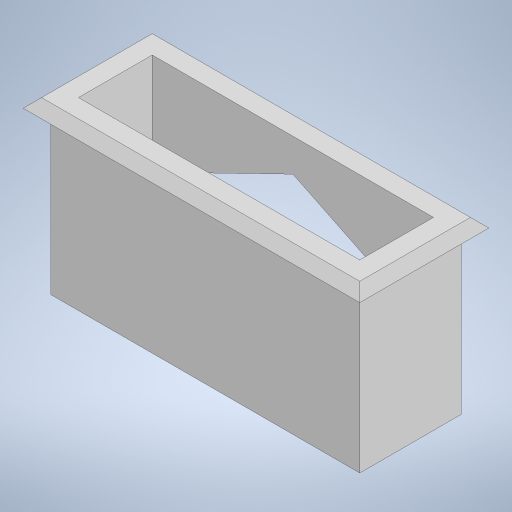
# Autodesk Inventor part: Controller Stand Breakout Holder
Saved by Autodesk Inventor 2024.1 (Build 281209000, 209)
## iProperties
Created: 2024-02-12
Part Number: Controller Stand Breakout Holder
Material: Generic
Document SubType Name: Modeling
Designer: ryanm
Density: 1 g/cm^3
Appearance: Default
Author: ryanm
Autodesk Inventor part; units mm, degrees
ref_plane "YZ Plane" through (0, 0, 0) normal (1, 0, 0) x (0, 1, 0)
ref_plane "XZ Plane" through (0, 0, 0) normal (0, 1, 0) x (-1, 0, 0)
ref_plane "XY Plane" through (0, 0, 0) normal (0, 0, 1) x (1, 0, 0)
sketch "Sketch1" plane through (0, 0, 0) normal (0, 1, 0) x (-1, 0, 0)
  line L0 (30.5, -8) -> (-30.5, -8)
  line L1 (-30.5, -8) -> (-30.5, 8)
  line L2 (-30.5, 8) -> (30.5, 8)
  line L3 (30.5, 8) -> (30.5, -8)
  line L4 (33.5, -11) -> (-33.5, -11)
  line L5 (-33.5, -11) -> (-33.5, 11)
  line L6 (-33.5, 11) -> (33.5, 11)
  line L7 (33.5, 11) -> (33.5, -11)
  point P0 (0, 0)
  point P1 (0, -8)
  point P2 (30.5, 0)
  dimension "d0" = 16
  dimension "d2" = 3
  dimension "d3" = 61
  constraints: 16 end point, 4 parallel, 2 midpoint, 2 perpendicular, 1 horizontal, 1 horizontal alignment, 1 vertical alignment, 3 other
  measures "d0" distance of L2.end L0.start
  measures "d2" distance between parallel lines of L3 L7
  measures "d3" distance of L0.start L0.end
extrude "Extrusion1" add sketch "Sketch1" along normal blind 35
sketch "Sketch2" plane through (0, 35, 0) normal (0, 1, 0) x (1, 0, 0)
  line L0 (-30.5, -8) -> (-30.5, 8) projected
  line L1 (30.5, -8) -> (-30.5, -8) projected
  line L2 (30.5, 8) -> (30.5, -8) projected
  line L3 (-30.5, 8) -> (30.5, 8) projected
  line L4 (-36.5, 14) -> (-36.5, -14)
  line L5 (-36.5, -14) -> (36.5, -14)
  line L6 (36.5, -14) -> (36.5, 14)
  line L7 (36.5, 14) -> (-36.5, 14)
  point P0 (0, 0)
  dimension "d6" = 6
  constraints: 8 end point, 3 other
  measures "d6" distance between parallel lines of L0 L4
extrude "Extrusion2" add sketch "Sketch2" along normal blind 2
chamfer "Chamfer1" distance 2 angle 45 4 edges at (0, 37, 14) (-36.5, 37, 0) (0, 37, -14) (36.5, 37, 0)
sketch "Sketch3" plane through (-30.5, 0, 8) normal (1, 0, 0) x (0, 0, -1)
  line L0 (19, 0) -> (-3, 0) projected
  line L1 (-3, 0) -> (-3, 35) projected
  line L2 (19, 35) -> (-3, 35) projected
  line L3 (19, 0) -> (19, 35) projected
  line L4 (0, 0) -> (2, 0)
  line L5 (2, 0) -> (2, 23)
  line L6 (2, 23) -> (0, 23)
  line L7 (0, 23) -> (0, 0)
  line L8 (4.5, 0) -> (6.5, 0)
  line L9 (6.5, 0) -> (6.5, 12)
  line L10 (6.5, 12) -> (4.5, 12)
  line L11 (4.5, 12) -> (4.5, 0)
  point P0 (8, 0)
  point P1 (2, 0)
  dimension "d12" = 2
  dimension "d13" = 3
  dimension "d14" = 23
  dimension "d28" = 12
  dimension "d29" = 2
  dimension "d30" = 2.5
  constraints: 16 end point, 4 parallel, 2 horizontal, 2 perpendicular, 2 point on line
  measures "d12" distance of L6.end L5.end
  measures "d13" distance between parallel lines of L1 L7
  measures "d14" distance of L4.end L5.end
  measures "d28" distance of L8.end L9.end
  measures "d29" distance of L9.end L10.end
  measures "d30" distance between parallel lines of L5 L11
extrude "Extrusion3" add sketch "Sketch3" along normal blind 2 contours L0 L11 L10 L9 | L0 L7 L6 L5
sketch "Sketch4" plane through (30.5, 0, -8) normal (-1, 0, 0) x (0, 0, 1)
  line L0 (19, 0) -> (-3, 0) projected
  line L1 (-3, 0) -> (-3, 35) projected
  line L2 (19, 35) -> (-3, 35) projected
  line L3 (19, 0) -> (19, 35) projected
  line L4 (14, 0) -> (16, 0)
  line L5 (16, 0) -> (16, 23)
  line L6 (16, 23) -> (14, 23)
  line L7 (14, 23) -> (14, 0)
  line L8 (11.5, 0) -> (9.5, 0)
  line L9 (9.5, 0) -> (9.5, 12)
  line L10 (9.5, 12) -> (11.5, 12)
  line L11 (11.5, 12) -> (11.5, 0)
  point P0 (8, 0)
  dimension "d20" = 2
  dimension "d21" = 23
  dimension "d22" = 3
  dimension "d31" = 2
  dimension "d32" = 12
  dimension "d33" = 2.5
  constraints: 16 end point, 4 parallel, 2 horizontal, 2 perpendicular, 2 point on line
  measures "d20" distance of L6.end L5.end
  measures "d21" distance of L6.end L4.start
  measures "d22" distance between parallel lines of L3 L5
  measures "d31" distance of L9.end L10.end
  measures "d32" distance of L8.end L9.end
  measures "d33" distance between parallel lines of L7 L11
extrude "Extrusion4" add sketch "Sketch4" along normal blind 2 contours L0 L7 L6 L5 | L0 L9 L10 L11
chamfer "Chamfer4" distance 2 angle 45 4 edges at (-29.5, 23, 6) (-29.5, 12, 3.5) (29.5, 12, 3.5) (29.5, 23, 6)
sketch "Sketch5" plane through (33.5, 0, -11) normal (0, 0, -1) x (-1, 0, 0)
  line L0 (0, 0) -> (67, 0) projected
  line L1 (67, 0) -> (67, 35) projected
  line L2 (3, 15) -> (33.5, 29.8758)
  line L3 (33.5, 29.8758) -> (64, 15)
  line L4 (0, 0) -> (0, 35) projected
  line L5 (3, 15) -> (64, 15) construction
  line L6 (3, 0) -> (3, 12) projected
  line L7 (3, 15) -> (3, 0)
  line L8 (64, 15) -> (64, 0)
  point P0 (33.5, 0)
  point P1 (33.5, 0)
  point P2 (33.5, 0)
  point P3 (33.5, 0)
  point P4 (33.5, 0)
  dimension "d40" = 3
  dimension "d41" = 3
  dimension "d42" = 26
  dimension "d43" = 15
  constraints: 10 end point, 1 horizontal, 1 horizontal alignment, 1 vertical, 1 vertical alignment, 6 other
  measures "d40" distance from line of L4 L2.start
  measures "d41" distance from line of L1 L3.end
  measures "d42" angle of L5 L2
  measures "d43" distance from line of point (33.5, 0) L5
extrude "Extrusion5" cut sketch "Sketch5" against normal up to surface (3 mm away)
equation "\"d41\" = d40"
body "Solid1"
